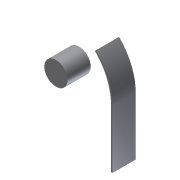
# Autodesk Inventor part: ShooterWheelrConcept
Saved by Autodesk Inventor 2012 (Build 160160000, 160)
## iProperties
Created: 2012-01-09
Part Number: ShooterWheelrConcept
Material: Default
Document SubType Name: Modeling
Designer: JesseK
Density: 1 g/cm^3
Author: JesseK
Autodesk Inventor part; units mm, degrees
ref_plane "YZ Plane" through (0, 0, 0) normal (1, 0, 0) x (0, 1, 0)
ref_plane "XZ Plane" through (0, 0, 0) normal (0, 1, 0) x (-1, 0, 0)
ref_plane "XY Plane" through (0, 0, 0) normal (0, 0, 1) x (1, 0, 0)
sketch "Sketch1" plane through (0, 0, 0) normal (0, 0, 1) x (1, 0, 0)
  arc A0 (241.3, 0) -> (170.6249, 170.6249) centre (0, 0) ccw
  arc A1 (247.65, 0) -> (175.115, 175.115) centre (0, 0) ccw
  line L0 (175.115, 175.115) -> (170.6249, 170.6249)
  line L1 (170.6249, 170.6249) -> (0, 0) construction
  circle A2 centre (0, 0) radius 50.8
  line L2 (241.3, 0) -> (241.3, -254)
  line L3 (241.3, -254) -> (247.65, -254)
  line L4 (247.65, -254) -> (247.65, 0)
  line L5 (241.3, 0) -> (247.65, 0) construction
  dimension "d0" = 241.3
  dimension "d1" = 247.65
  dimension "d3" = 101.6
  dimension "d4" = 254
  dimension "d5" = 45
  constraints: 12 end point, 5 point on circle, 3 centre point, 3 coincident, 2 perpendicular, 2 tangent, 1 collinear, 1 parallel, 1 vertical
  measures "d0" radius of A0
  measures "d1" radius of A1
  measures "d3" diameter of A2
  measures "d4" distance of L2.start L2.end
  measures "d5" angle of L1 L5
extrude "Extrusion1" add sketch "Sketch1" along normal blind 101.6
body "Solid1"
